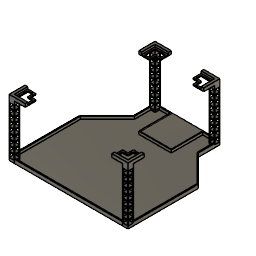
Maze solver chassis (Autodesk Fusion 360 design; units mm, degrees)
Autodesk Fusion 360 part; units mm, degrees
sketch "Sketch1" plane through (0, 0, 0) normal (0, 0, 1) x (1, 0, 0)
  line L0 (0, 0) -> (100, 0)
  line L1 (100, 0) -> (100, 60)
  line L2 (0, 0) -> (0, 60)
  line L3 (0, 60) -> (25, 85)
  line L4 (100, 60) -> (75, 85)
  line L5 (25, 85) -> (25, 100)
  line L6 (25, 100) -> (75, 100)
  line L7 (75, 100) -> (75, 85)
  line L8 (100, -5) -> (-5, -5)
  line L9 (-5, -5) -> (-5, 60)
  line L10 (105, 60) -> (105, -5)
  line L11 (105, -5) -> (100, -5)
  line L12 (25, 105) -> (75, 105)
  line L13 (75, 105) -> (80, 105)
  line L14 (80, 105) -> (80, 85)
  line L15 (80, 85) -> (105, 60)
  line L16 (25, 105) -> (20, 105)
  line L17 (20, 105) -> (20, 85)
  line L18 (20, 85) -> (-5, 60)
  line L19 (0, 0) -> (5, 0)
  line L20 (5, 5) -> (95, 5)
  line L21 (95, 5) -> (95, 60)
  line L22 (5, 60) -> (5, 5)
  line L23 (30, 95) -> (70, 95)
  line L24 (70, 95) -> (70, 85)
  line L25 (70, 85) -> (95, 60)
  line L26 (30, 95) -> (30, 85)
  line L27 (30, 85) -> (5, 60)
  dimension "d2" = 60
  dimension "d3" = 60
  dimension "d8" = 50
  dimension "d10" = 5
  dimension "d11" = 105
  dimension "d12" = 65
  dimension "d13" = 110
  constraint coincident L0.start L2.start
  constraint horizontal L0
  constraint coincident L0 L19.end
  measures "d2" distance of L0.end L1.end
  measures "d3" distance of L0.start L2.end
  measures "d8" distance of L5.end L6.end
  measures "d10" distance of L0.end L8.start
  measures "d11" distance of L8.start L8.end
  measures "d12" distance of L8.end L9.end
  measures "d13" distance of L9.end L10.start
sketch "Sketch2" plane through (0, 0, 0) normal (0, 0, 1) x (1, 0, 0)
  line L0 (102.5, 10) -> (105, 10)
  line L1 (105, 10) -> (105, -5)
  line L2 (105, -5) -> (90, -5)
  line L3 (90, -5) -> (90, -2.5)
  line L4 (-5, -5) -> (10, -5)
  line L5 (10, -5) -> (10, -2.5)
  line L6 (-2.5, 10) -> (-5, 10)
  line L7 (-5, 10) -> (-5, -5)
  line L8 (65, 102.5) -> (65, 105)
  line L9 (65, 105) -> (80, 105)
  line L10 (80, 105) -> (80, 90)
  line L11 (80, 90) -> (77.5, 90)
  line L12 (35, 102.5) -> (35, 105)
  line L13 (35, 105) -> (20, 105)
  line L14 (20, 105) -> (20, 95)
  line L15 (20, 95) -> (20, 90)
  line L16 (20, 90) -> (22.5, 90)
  line L17 (20, 90) -> (22.5, 90)
  line L18 (20, 90) -> (22.5, 90)
  line L19 (22.5, 90) -> (22.5, 102.5)
  line L20 (35, 102.5) -> (22.5, 102.5)
  line L21 (65, 102.5) -> (77.5, 102.5)
  line L22 (77.5, 102.5) -> (77.5, 90)
  line L23 (102.5, 10) -> (102.5, -2.5)
  line L24 (102.5, -2.5) -> (90, -2.5)
  line L25 (10, -2.5) -> (-2.5, -2.5)
  line L26 (-2.5, -2.5) -> (-2.5, 10)
  line L27 (35, 102.5) -> (35, 95)
  line L28 (30, 95) -> (35, 95)
  line L29 (30, 95) -> (30, 90)
  line L30 (30, 90) -> (22.5, 90)
  line L31 (65, 102.5) -> (65, 95)
  line L32 (65, 95) -> (70, 95)
  line L33 (70, 95) -> (70, 90)
  line L34 (70, 90) -> (77.5, 90)
  line L35 (102.5, 10) -> (95, 10)
  line L36 (95, 10) -> (95, 5)
  line L37 (95, 5) -> (90, 5)
  line L38 (90, 5) -> (90, -2.5)
  line L39 (-2.5, 10) -> (5, 10)
  line L40 (5, 10) -> (5, 5)
  line L41 (5, 5) -> (10, 5)
  line L42 (10, 5) -> (10, -2.5)
  line L43 (90, 5) -> (90, 3.5)
  line L44 (91.5, 3.5) -> (95, 3.5)
  line L45 (95, 5) -> (95, 10)
  line L46 (95, 10) -> (96.5, 10)
  line L47 (96.5, 8.5) -> (96.5, 3.5)
  line L48 (96.5, 3.5) -> (95, 3.5)
  line L49 (91.5, 3.5) -> (91.5, -1)
  line L50 (91.5, -1) -> (101, -1)
  line L51 (101, -1) -> (101, 8.5)
  line L52 (101, 8.5) -> (96.5, 8.5)
  line L53 (10, 5) -> (10, 3.5)
  line L54 (8.5, 3.5) -> (3.5, 3.5)
  line L55 (3.5, 3.5) -> (3.5, 8.5)
  line L56 (3.5, 8.5) -> (-1, 8.5)
  line L57 (-1, 8.5) -> (-1, -1)
  line L58 (-1, -1) -> (8.5, -1)
  line L59 (8.5, -1) -> (8.5, 3.5)
  line L60 (35, 102.5) -> (35, 101)
  line L61 (33.5, 101) -> (24, 101)
  line L62 (24, 101) -> (24, 91.5)
  line L63 (24, 91.5) -> (28.5, 91.5)
  line L64 (28.5, 91.5) -> (28.5, 96.5)
  line L65 (28.5, 96.5) -> (33.5, 96.5)
  line L66 (33.5, 96.5) -> (33.5, 101)
  line L67 (65, 102.5) -> (65, 101)
  line L68 (66.5, 101) -> (76, 101)
  line L69 (76, 101) -> (76, 91.5)
  line L70 (76, 91.5) -> (71.5, 91.5)
  line L71 (71.5, 91.5) -> (71.5, 96.5)
  line L72 (71.5, 96.5) -> (66.5, 96.5)
  line L73 (66.5, 96.5) -> (66.5, 101)
  dimension "d16" = 15
  dimension "d17" = 15
  constraint coincident L38 L43.end
  constraint coincident L35 L46.end
  constraint coincident L42 L53.end
  constraint coincident L31 L67.end
  measures "d16" distance of L4.start L4.end
  measures "d17" distance of L9.end L10.end
sketch "Sketch3" plane through (0, 0, 0) normal (0, 0, 1) x (1, 0, 0)
  line L0 (100, -5) -> (100, 0)
  line L1 (100, 0) -> (105, 0)
  line L2 (105, 0) -> (105, -5)
  line L3 (105, -5) -> (100, -5)
  line L4 (75, 100) -> (75, 105)
  line L5 (75, 105) -> (80, 105)
  line L6 (80, 105) -> (80, 100)
  line L7 (80, 100) -> (75, 100)
  line L8 (25, 100) -> (25, 105)
  line L9 (25, 105) -> (20, 105)
  line L10 (20, 105) -> (20, 100)
  line L11 (20, 100) -> (25, 100)
  line L12 (-5, -5) -> (0, -5)
  line L13 (0, -5) -> (0, 0)
  line L14 (0, 0) -> (-5, 0)
  line L15 (-5, 0) -> (-5, -5)
  constraint vertical L0
  constraint perpendicular L0 L1
  constraint perpendicular L1 L2
  constraint perpendicular L0 L3
  constraint perpendicular L1 L4
  constraint perpendicular L4 L5
  constraint perpendicular L5 L6
  constraint perpendicular L4 L7
  constraint perpendicular L5 L8
  constraint perpendicular L4 L9
  constraint perpendicular L9 L10
  constraint perpendicular L4 L11
  constraint perpendicular L4 L12
  constraint coincident L13.end L14.start
  constraint perpendicular L9 L13
  constraint perpendicular L13 L14
  constraint perpendicular L12 L15
sketch "Sketch4" plane through (0, 0, 0) normal (0, 0, 1) x (1, 0, 0)
  line L0 (-5, -5, -50) -> (-5, 105, -50)
  line L1 (-5, 105, -50) -> (105, 105, -50)
  line L2 (105, 105, -50) -> (105, -5, -50)
  line L3 (105, -5, -50) -> (-5, -5, -50)
extrude "Extrude1" add sketch "Sketch2" along normal blind 1 contours L0 L1 L2 L3 L23 L24 | L23 L24 L35 L36 L37 L38 L43 L45 L46 | L4 L5 L6 L7 L25 L26 | L25 L26 L39 L40 L41 L42 L53 | L8 L9 L10 L11 L21 L22 | L21 L22 L31 L32 L33 L34 L67 | L12 L13 L14 L15 L16 L17 L18 L19 L20 | L19 L20 L27 L28 L29 L30 L60 | L44 L47 L48 L49 L50 L51 L52 | L54 L55 L56 L57 L58 L59 | L61 L62 L63 L64 L65 L66 | L68 L69 L70 L71 L72 L73 makes body 1 at (-1.6667, 3.3333, 0) makes body 2 at (28.3333, 101.6667, 0) makes body 3 at (96.6667, -1.6667, 0) makes body 4 at (71.6667, 101.6667, 0)
extrude "Extrude2" add sketch "Sketch2" along normal blind 3 contours L0 L1 L2 L3 L23 L24 | L4 L5 L6 L7 L25 L26 | L8 L9 L10 L11 L21 L22 | L12 L13 L14 L15 L16 L17 L18 L19 L20 bodies 1 2 3 4
extrude "Extrude3" add sketch "Sketch3" against normal blind 50 bodies 1 2 3 4
extrude "Extrude4" add sketch "Sketch4" along normal blind 1 contours L0 L1 L2 L3 in plane through (0, 0, -50) normal (0, 0, 1) bodies 1 2 3 4
sketch "Sketch5" plane through (0, 0, 0) normal (0, 0, 1) x (1, 0, 0)
  line L0 (20, 85, -50) -> (-5, 60, -50)
  line L1 (20, 105, -50) -> (20, 85, -50)
  line L2 (25, 105, -50) -> (20, 105, -50)
  line L3 (25, 105, -50) -> (75, 105, -50)
  line L4 (75, 105, -50) -> (80, 105, -50)
  line L5 (80, 105, -50) -> (80, 85, -50)
  line L6 (80, 85, -50) -> (105, 60, -50)
  line L7 (105, 60, -50) -> (105, -5, -50)
  line L8 (105, -5, -50) -> (100, -5, -50)
  line L9 (100, -5, -50) -> (-5, -5, -50)
  line L10 (-5, -5, -50) -> (-5, 60, -50)
  dimension "d27" = 105
  dimension "d28" = 65
  dimension "d29" = 110
ref_plane "WorkPlane1" through (50, 50, -50) normal (0, 0, 1) x (1, 0, 0)
sketch "Sketch6" plane through (0, 0, -50) normal (0, 0, 1) x (1, 0, 0)
  line L0 (-5, 60) -> (-5, 105)
  line L1 (-5, 105) -> (20, 105)
  line L2 (20, 105) -> (20, 85)
  line L3 (20, 85) -> (-5, 60)
  line L4 (80, 105) -> (105, 105)
  line L5 (105, 105) -> (105, 60)
  line L6 (105, 60) -> (80, 85)
  line L7 (80, 85) -> (80, 105)
  constraint vertical L0
  constraint perpendicular L0 L1
  constraint perpendicular L1 L2
  constraint perpendicular L0 L4
  constraint perpendicular L4 L5
  constraint perpendicular L3 L6
  constraint perpendicular L4 L7
extrude "Extrude5" cut sketch "Sketch6" along normal blind 1 bodies 1
sketch "Sketch7" plane through (0, 0, -50) normal (0, 0, 1) x (1, 0, 0)
  line L0 (50, 105) -> (65, 105)
  line L1 (65, 105) -> (65, 75)
  line L2 (65, 75) -> (35, 75)
  line L3 (35, 75) -> (35, 105)
  line L4 (35, 105) -> (50, 105)
  dimension "d33" = 15
  dimension "d34" = 30
  dimension "d35" = 30
  dimension "d36" = 30
  constraint horizontal L0
  constraint perpendicular L0 L1
  constraint perpendicular L1 L2
  constraint perpendicular L0 L3
  measures "d33" distance of L0.start L0.end
  measures "d34" distance of L0.end L1.end
  measures "d35" distance of L1.end L2.end
  measures "d36" distance of L2.end L3.end
extrude "Extrude6" add sketch "Sketch7" along normal blind 10 bodies 1
extrude "Extrude7" cut sketch "Sketch7" along normal blind 9 bodies 1 makes body 5 at (45, 95, -41)
sketch "Sketch8" plane through (0, 0, -50) normal (0, 0, 1) x (1, 0, 0)
  line L0 (35, 105) -> (36, 105)
  line L1 (36, 105) -> (36, 76)
  line L2 (36, 76) -> (64, 76)
  line L3 (64, 76) -> (64, 105)
  line L4 (35, 105) -> (36, 105)
  line L5 (64, 105) -> (65, 105)
  line L6 (36, 105) -> (35, 105)
  line L7 (35, 105) -> (35, 75)
  line L8 (35, 75) -> (65, 75)
  line L9 (65, 75) -> (65, 105)
  line L10 (64, 105) -> (36, 105)
  constraint perpendicular L1 L6
  constraint perpendicular L6 L7
  constraint perpendicular L1 L8
  constraint perpendicular L5 L9
  constraint perpendicular L1 L10
extrude "Extrude8" add sketch "Sketch8" along normal blind 10 contours L0 L1 L2 L3 L4 L5 L6 L7 L8 L9 bodies 1 5
sketch "Sketch9" plane through (0, 0, 0) normal (1, 0, 0) x (0, 1, 0)
  line L0 (10, -50) -> (10, -65)
  circle A0 centre (10, -57.5) radius 25
  line L1 (10, -82.5) -> (100, -82.5)
  line L2 (100, -82.5) -> (100, -47.5)
  line L3 (105, -50) -> (105, -47.5)
  line L4 (105, -47.5) -> (75, -47.5)
  dimension "d43" = 15
  dimension "d45" = 35
  dimension "d46" = 2.5
  dimension "d47" = 30
  constraint coincident A0 L1.start
  constraint tangent A0 L1
  constraint perpendicular L0 L1
  constraint perpendicular L1 L2
  constraint vertical L3
  constraint perpendicular L3 L4
  measures "d43" distance of L0.start L0.end
  measures "d45" distance of L1.end L2.end
  measures "d46" distance of L3.start L3.end
  measures "d47" distance of L3.end L4.end
sketch "Sketch10" plane through (0, 105, 0) normal (0, 1, 0) x (-1, 0, 0)
  line L0 (-65, -49) -> (-75, -49)
  line L1 (-75, -49) -> (-75, 0)
  line L2 (-75, 0) -> (-65, 0)
  line L3 (-65, 0) -> (-65, 3)
  line L4 (-65, 3) -> (-80, 3)
  line L5 (-80, 3) -> (-80, -50)
  line L6 (-80, -50) -> (-64, -50)
  line L7 (-64, -50) -> (-64, -41)
  line L8 (-64, -41) -> (-36, -41)
  line L9 (-36, -41) -> (-36, -50)
  line L10 (-36, -50) -> (-20, -50)
  line L11 (-20, -50) -> (-20, 3)
  line L12 (-20, 3) -> (-35, 3)
  line L13 (-35, 3) -> (-35, 0)
  line L14 (-35, 0) -> (-25, 0)
  line L15 (-25, 0) -> (-25, -49)
  line L16 (-25, -49) -> (-35, -49)
  line L17 (-35, -49) -> (-35, -40)
  line L18 (-35, -40) -> (-65, -40)
  line L19 (-65, -40) -> (-65, -49)
  line L20 (0, -47.5) -> (-100, -47.5)
  constraint perpendicular L5 L20
extrude "Extrude9" cut 1 faces at (45, 95, -40) along direction (0, 0, -1) blind 7.5 on bodies 1 bodies 1
extrude "Extrude10" add sketch "Sketch7" along normal blind 3.5 bodies 1
extrude "Extrude11" cut sketch "Sketch8" along normal blind 3 contours L1 L2 L3 L10 bodies 1
extrude "Extrude12" cut sketch "Sketch2" along normal blind 2 contours L44 L47 L48 L49 L50 L51 L52 | L54 L55 L56 L57 L58 L59 | L61 L62 L63 L64 L65 L66 | L68 L69 L70 L71 L72 L73 bodies 1
sketch "Sketch11" plane through (-5, 0, 0) normal (-1, 0, 0) x (0, -1, 0)
  line L0 (-60, -49) -> (-60, -50)
  line L1 (-60, -50) -> (5, -50)
  line L2 (5, -50) -> (5, 3)
  line L3 (5, 3) -> (-10, 3)
  line L4 (-10, 3) -> (-10, 0)
  line L5 (-10, 0) -> (0, 0)
  line L6 (0, 0) -> (0, -49)
  line L7 (0, -49) -> (-60, -49)
  line L8 (5, -50) -> (2.5, -50)
  line L9 (4.5, -47.5) -> (0.5, -47.5)
  line L10 (0.5, -47.5) -> (0.5, -43.5)
  line L11 (0.5, -43.5) -> (4.5, -43.5)
  line L12 (4.5, -43.5) -> (4.5, -47.5)
  line L13 (4.5, -47.5) -> (0.5, -43.5) construction
  line L14 (0.5, -38.5) -> (4.5, -38.5)
  line L15 (0.5, -42.5) -> (0.5, -38.5)
  line L16 (4.5, -42.5) -> (0.5, -38.5) construction
  line L17 (4.5, -38.5) -> (4.5, -42.5)
  line L18 (4.5, -42.5) -> (0.5, -42.5)
  line L19 (4.5, -32.5) -> (0.5, -32.5)
  line L20 (0.5, -28.5) -> (4.5, -28.5)
  line L21 (4.5, -28.5) -> (4.5, -32.5)
  line L22 (4.5, -37.5) -> (0.5, -37.5)
  line L23 (4.5, -32.5) -> (0.5, -28.5) construction
  line L24 (0.5, -33.5) -> (4.5, -33.5)
  line L25 (4.5, -33.5) -> (4.5, -37.5)
  line L26 (0.5, -32.5) -> (0.5, -28.5)
  line L27 (0.5, -37.5) -> (0.5, -33.5)
  line L28 (4.5, -37.5) -> (0.5, -33.5) construction
  line L29 (4.5, -22.5) -> (0.5, -22.5)
  line L30 (0.5, -17.5) -> (0.5, -13.5)
  line L31 (0.5, -27.5) -> (0.5, -23.5)
  line L32 (4.5, -12.5) -> (0.5, -8.5) construction
  line L33 (0.5, -13.5) -> (4.5, -13.5)
  line L34 (0.5, -12.5) -> (0.5, -8.5)
  line L35 (4.5, -12.5) -> (0.5, -12.5)
  line L36 (0.5, -8.5) -> (4.5, -8.5)
  line L37 (0.5, -18.5) -> (4.5, -18.5)
  line L38 (4.5, -17.5) -> (0.5, -17.5)
  line L39 (4.5, -27.5) -> (0.5, -23.5) construction
  line L40 (5, -30) -> (2.5, -30)
  line L41 (0.5, -22.5) -> (0.5, -18.5)
  line L42 (4.5, -18.5) -> (4.5, -22.5)
  line L43 (4.5, -23.5) -> (4.5, -27.5)
  line L44 (4.5, -27.5) -> (0.5, -27.5)
  line L45 (4.5, -22.5) -> (0.5, -18.5) construction
  line L46 (0.5, -23.5) -> (4.5, -23.5)
  line L47 (4.5, -13.5) -> (4.5, -17.5)
  line L48 (4.5, -8.5) -> (4.5, -12.5)
  line L49 (4.5, -17.5) -> (0.5, -13.5) construction
  line L50 (0.5, -7.5) -> (0.5, -3.5)
  line L51 (4.5, -7.5) -> (0.5, -7.5)
  line L52 (4.5, -7.5) -> (0.5, -3.5) construction
  line L53 (4.5, -3.5) -> (4.5, -7.5)
  line L54 (0.5, -3.5) -> (4.5, -3.5)
  line L55 (0.5, -23.5) -> (4.5, -23.5)
  line L56 (0.5, -13.5) -> (4.5, -13.5)
  line L57 (4.5, -38.5) -> (4.5, -42.5)
  line L58 (4.5, -3.5) -> (4.5, -7.5)
  line L59 (4.5, -43.5) -> (4.5, -47.5)
  line L60 (0.5, -7.5) -> (0.5, -3.5)
  line L61 (4.5, -7.5) -> (0.5, -3.5) construction
  line L62 (4.5, -22.5) -> (0.5, -22.5)
  line L63 (4.5, -47.5) -> (0.5, -47.5)
  line L64 (4.5, -12.5) -> (0.5, -8.5) construction
  line L65 (4.5, -12.5) -> (0.5, -12.5)
  line L66 (0.5, -42.5) -> (0.5, -38.5)
  line L67 (4.5, -32.5) -> (0.5, -32.5)
  line L68 (4.5, -42.5) -> (0.5, -42.5)
  line L69 (4.5, -42.5) -> (0.5, -38.5) construction
  line L70 (0.5, -47.5) -> (0.5, -43.5)
  line L71 (5, -50) -> (2.5, -50)
  line L72 (4.5, -28.5) -> (4.5, -32.5)
  line L73 (0.5, -43.5) -> (4.5, -43.5)
  line L74 (0.5, -37.5) -> (0.5, -33.5)
  line L75 (0.5, -3.5) -> (4.5, -3.5)
  line L76 (4.5, -7.5) -> (0.5, -7.5)
  line L77 (0.5, -8.5) -> (4.5, -8.5)
  line L78 (4.5, -47.5) -> (0.5, -43.5) construction
  line L79 (4.5, -8.5) -> (4.5, -12.5)
  line L80 (0.5, -12.5) -> (0.5, -8.5)
  line L81 (0.5, -38.5) -> (4.5, -38.5)
  line L82 (0.5, -18.5) -> (4.5, -18.5)
  line L83 (0.5, -22.5) -> (0.5, -18.5)
  line L84 (4.5, -33.5) -> (4.5, -37.5)
  line L85 (4.5, -23.5) -> (4.5, -27.5)
  line L86 (0.5, -28.5) -> (4.5, -28.5)
  line L87 (4.5, -37.5) -> (0.5, -37.5)
  line L88 (4.5, -18.5) -> (4.5, -22.5)
  line L89 (4.5, -27.5) -> (0.5, -27.5)
  line L90 (0.5, -32.5) -> (0.5, -28.5)
  line L91 (4.5, -32.5) -> (0.5, -28.5) construction
  line L92 (4.5, -27.5) -> (0.5, -23.5) construction
  line L93 (4.5, -22.5) -> (0.5, -18.5) construction
  line L94 (4.5, -17.5) -> (0.5, -17.5)
  line L95 (4.5, -37.5) -> (0.5, -33.5) construction
  line L96 (5, -30) -> (2.5, -30)
  line L97 (0.5, -33.5) -> (4.5, -33.5)
  line L98 (0.5, -27.5) -> (0.5, -23.5)
  line L99 (4.5, -13.5) -> (4.5, -17.5)
  line L100 (0.5, -17.5) -> (0.5, -13.5)
  line L101 (4.5, -17.5) -> (0.5, -13.5) construction
  line L102 (-104.5, -23.5) -> (-100.5, -23.5)
  line L103 (-104.5, -13.5) -> (-100.5, -13.5)
  line L104 (-100.5, -38.5) -> (-100.5, -42.5)
  line L105 (-100.5, -3.5) -> (-100.5, -7.5)
  line L106 (-100.5, -43.5) -> (-100.5, -47.5)
  line L107 (-104.5, -7.5) -> (-104.5, -3.5)
  line L108 (-100.5, -7.5) -> (-104.5, -3.5) construction
  line L109 (-100.5, -22.5) -> (-104.5, -22.5)
  line L110 (-100.5, -47.5) -> (-104.5, -47.5)
  line L111 (-100.5, -12.5) -> (-104.5, -8.5) construction
  line L112 (-100.5, -12.5) -> (-104.5, -12.5)
  line L113 (-104.5, -42.5) -> (-104.5, -38.5)
  line L114 (-100.5, -32.5) -> (-104.5, -32.5)
  line L115 (-100.5, -42.5) -> (-104.5, -42.5)
  line L116 (-100.5, -42.5) -> (-104.5, -38.5) construction
  line L117 (-104.5, -47.5) -> (-104.5, -43.5)
  line L118 (-100, -50) -> (-102.5, -50)
  line L119 (-100.5, -28.5) -> (-100.5, -32.5)
  line L120 (-104.5, -43.5) -> (-100.5, -43.5)
  line L121 (-104.5, -37.5) -> (-104.5, -33.5)
  line L122 (-104.5, -3.5) -> (-100.5, -3.5)
  line L123 (-100.5, -7.5) -> (-104.5, -7.5)
  line L124 (-104.5, -8.5) -> (-100.5, -8.5)
  line L125 (-100.5, -47.5) -> (-104.5, -43.5) construction
  line L126 (-100.5, -8.5) -> (-100.5, -12.5)
  line L127 (-104.5, -12.5) -> (-104.5, -8.5)
  line L128 (-104.5, -38.5) -> (-100.5, -38.5)
  line L129 (-104.5, -18.5) -> (-100.5, -18.5)
  line L130 (-104.5, -22.5) -> (-104.5, -18.5)
  line L131 (-100.5, -33.5) -> (-100.5, -37.5)
  line L132 (-100.5, -23.5) -> (-100.5, -27.5)
  line L133 (-104.5, -28.5) -> (-100.5, -28.5)
  line L134 (-100.5, -37.5) -> (-104.5, -37.5)
  line L135 (-100.5, -18.5) -> (-100.5, -22.5)
  line L136 (-100.5, -27.5) -> (-104.5, -27.5)
  line L137 (-104.5, -32.5) -> (-104.5, -28.5)
  line L138 (-100.5, -32.5) -> (-104.5, -28.5) construction
  line L139 (-100.5, -27.5) -> (-104.5, -23.5) construction
  line L140 (-100.5, -22.5) -> (-104.5, -18.5) construction
  line L141 (-100.5, -17.5) -> (-104.5, -17.5)
  line L142 (-100.5, -37.5) -> (-104.5, -33.5) construction
  line L143 (-100, -30) -> (-102.5, -30)
  line L144 (-104.5, -33.5) -> (-100.5, -33.5)
  line L145 (-104.5, -27.5) -> (-104.5, -23.5)
  line L146 (-100.5, -13.5) -> (-100.5, -17.5)
  line L147 (-104.5, -17.5) -> (-104.5, -13.5)
  line L148 (-100.5, -17.5) -> (-104.5, -13.5) construction
  point P0 (2.5, -45.5)
  point P1 (2.5, -40.5)
  point P2 (2.5, -30.5)
  point P3 (2.5, -35.5)
  point P4 (2.5, -20.5)
  point P5 (2.5, -10.5)
  point P6 (2.5, -15.5)
  point P7 (2.5, -25.5)
  point P8 (0, -29)
  point P9 (2.5, -5.5)
  point P10 (2.5, -5.5)
  point P11 (2.5, -40.5)
  point P12 (2.5, -20.5)
  point P13 (2.5, -30.5)
  point P14 (2.5, -35.5)
  point P15 (2.5, -15.5)
  point P16 (2.5, -25.5)
  point P17 (0, -29)
  point P18 (2.5, -10.5)
  point P19 (2.5, -45.5)
  point P20 (5, -50)
  point P21 (0, -49)
  point P22 (-102.5, -5.5)
  point P23 (-102.5, -40.5)
  point P24 (-102.5, -20.5)
  point P25 (-102.5, -30.5)
  point P26 (-102.5, -35.5)
  point P27 (-102.5, -15.5)
  point P28 (-102.5, -25.5)
  point P29 (-105, -29)
  point P30 (-102.5, -10.5)
  point P31 (-102.5, -45.5)
  point P32 (-100, -50)
  point P33 (-105, -49)
  dimension "d74" = 2.5
  dimension "d79" = 2.5
  dimension "d80" = 2.5
  dimension "d81" = 2.5
  dimension "d82" = 2.5
  dimension "d83" = 2.5
  constraint coincident P20 L1.end
  constraint coincident L1 L8.end
  constraint horizontal L9
  constraint coincident L13 P19
  constraint horizontal L18
  constraint coincident P11 L16
  constraint horizontal L22
  constraint coincident P14 L28
  constraint horizontal L19
  constraint coincident P13 L23
  constraint horizontal L44
  constraint coincident P16 L39
  constraint horizontal L29
  constraint coincident P12 L45
  constraint horizontal L38
  constraint coincident P15 L49
  constraint horizontal L35
  constraint coincident P18 L32
  constraint horizontal L51
  constraint coincident P10 L52
  constraint horizontal L63
  constraint coincident P19 L78
  constraint horizontal L68
  constraint coincident P11 L69
  constraint horizontal L87
  constraint coincident P14 L95
  constraint horizontal L67
  constraint coincident P13 L91
  constraint horizontal L89
  constraint coincident P16 L92
  constraint horizontal L62
  constraint coincident P12 L93
  constraint horizontal L94
  constraint coincident P15 L101
  constraint horizontal L65
  constraint coincident P18 L64
  constraint horizontal L76
  constraint coincident P10 L61
  constraint coincident P32 L118.start
  constraint horizontal L110
  constraint coincident P31 L125
  constraint horizontal L115
  constraint coincident P23 L116
  constraint horizontal L134
  constraint coincident P26 L142
  constraint horizontal L114
  constraint coincident P25 L138
  constraint horizontal L136
  constraint coincident P28 L139
  constraint horizontal L109
  constraint coincident P24 L140
  constraint horizontal L141
  constraint coincident P27 L148
  constraint horizontal L112
  constraint coincident P30 L111
  constraint horizontal L123
  constraint coincident P22 L108
  measures "d74" distance of P20 L8.end
  measures "d79" distance of L40.start L40.end
  measures "d80" distance of P20 L8.end
  measures "d81" distance of L40.start L40.end
  measures "d82" distance of P32 L118.end
  measures "d83" distance of L143.start L143.end
extrude "Extrude13" cut sketch "Sketch11" against normal blind 120 contours L9 L10 L11 L12 L59 L63 L70 L73 | L14 L15 L17 L18 L57 L66 L68 L81 | L19 L20 L21 L26 L67 L72 L86 L90 | L22 L24 L25 L27 L74 L84 L87 L97 | L29 L37 L41 L42 L62 L82 L83 L88 | L30 L33 L38 L47 L56 L94 L99 L100 | L31 L43 L44 L46 L55 L85 L89 L98 | L34 L35 L36 L48 L65 L77 L79 L80 | L50 L51 L53 L54 L58 L60 L75 L76 | L102 L132 L136 L145 | L103 L141 L146 L147 | L104 L113 L115 L128 | L105 L107 L122 L123 | L109 L129 L130 L135 | L112 L124 L126 L127 | L114 L119 L133 L137 | L121 L131 L134 L144 bodies 1
sketch "Sketch12" plane through (0, -5, 0) normal (0, -1, 0) x (1, 0, 0)
  line L0 (0, -49) -> (0, 0)
  line L1 (0, 0) -> (10, 0)
  line L2 (10, 0) -> (10, 3)
  line L3 (10, 3) -> (-5, 3)
  line L4 (-5, 3) -> (-5, -50)
  line L5 (-5, -50) -> (0, -50)
  line L6 (0, -50) -> (0, -49)
  line L7 (-4.5, -23.5) -> (-0.5, -23.5)
  line L8 (-4.5, -13.5) -> (-0.5, -13.5)
  line L9 (-0.5, -38.5) -> (-0.5, -42.5)
  line L10 (-0.5, -3.5) -> (-0.5, -7.5)
  line L11 (-0.5, -43.5) -> (-0.5, -47.5)
  line L12 (-4.5, -7.5) -> (-4.5, -3.5)
  line L13 (-0.5, -7.5) -> (-4.5, -3.5) construction
  line L14 (-0.5, -22.5) -> (-4.5, -22.5)
  line L15 (-0.5, -47.5) -> (-4.5, -47.5)
  line L16 (-0.5, -12.5) -> (-4.5, -8.5) construction
  line L17 (-0.5, -12.5) -> (-4.5, -12.5)
  line L18 (-4.5, -42.5) -> (-4.5, -38.5)
  line L19 (-0.5, -32.5) -> (-4.5, -32.5)
  line L20 (-0.5, -42.5) -> (-4.5, -42.5)
  line L21 (-0.5, -42.5) -> (-4.5, -38.5) construction
  line L22 (-4.5, -47.5) -> (-4.5, -43.5)
  line L23 (0, -50) -> (-2.5, -50)
  line L24 (-0.5, -28.5) -> (-0.5, -32.5)
  line L25 (-4.5, -43.5) -> (-0.5, -43.5)
  line L26 (-4.5, -37.5) -> (-4.5, -33.5)
  line L27 (-4.5, -3.5) -> (-0.5, -3.5)
  line L28 (-0.5, -7.5) -> (-4.5, -7.5)
  line L29 (-4.5, -8.5) -> (-0.5, -8.5)
  line L30 (-0.5, -47.5) -> (-4.5, -43.5) construction
  line L31 (-0.5, -8.5) -> (-0.5, -12.5)
  line L32 (-4.5, -12.5) -> (-4.5, -8.5)
  line L33 (-4.5, -38.5) -> (-0.5, -38.5)
  line L34 (-4.5, -18.5) -> (-0.5, -18.5)
  line L35 (-4.5, -22.5) -> (-4.5, -18.5)
  line L36 (-0.5, -33.5) -> (-0.5, -37.5)
  line L37 (-0.5, -23.5) -> (-0.5, -27.5)
  line L38 (-4.5, -28.5) -> (-0.5, -28.5)
  line L39 (-0.5, -37.5) -> (-4.5, -37.5)
  line L40 (-0.5, -18.5) -> (-0.5, -22.5)
  line L41 (-0.5, -27.5) -> (-4.5, -27.5)
  line L42 (-4.5, -32.5) -> (-4.5, -28.5)
  line L43 (-0.5, -32.5) -> (-4.5, -28.5) construction
  line L44 (-0.5, -27.5) -> (-4.5, -23.5) construction
  line L45 (-0.5, -22.5) -> (-4.5, -18.5) construction
  line L46 (-0.5, -17.5) -> (-4.5, -17.5)
  line L47 (-0.5, -37.5) -> (-4.5, -33.5) construction
  line L48 (0, -30) -> (-2.5, -30)
  line L49 (-4.5, -33.5) -> (-0.5, -33.5)
  line L50 (-4.5, -27.5) -> (-4.5, -23.5)
  line L51 (-0.5, -13.5) -> (-0.5, -17.5)
  line L52 (-4.5, -17.5) -> (-4.5, -13.5)
  line L53 (-0.5, -17.5) -> (-4.5, -13.5) construction
  point P0 (-2.5, -5.5)
  point P1 (-2.5, -40.5)
  point P2 (-2.5, -20.5)
  point P3 (-2.5, -30.5)
  point P4 (-2.5, -35.5)
  point P5 (-2.5, -15.5)
  point P6 (-2.5, -25.5)
  point P7 (-5, -29)
  point P8 (-2.5, -10.5)
  point P9 (-2.5, -45.5)
  point P10 (0, -50)
  point P11 (-5, -49)
  dimension "d86" = 2.5
  dimension "d87" = 2.5
  constraint coincident P10 L5.end
  constraint horizontal L15
  constraint coincident P9 L30
  constraint horizontal L20
  constraint coincident P1 L21
  constraint horizontal L39
  constraint coincident P4 L47
  constraint horizontal L19
  constraint coincident P3 L43
  constraint horizontal L41
  constraint coincident P6 L44
  constraint horizontal L14
  constraint coincident P2 L45
  constraint horizontal L46
  constraint coincident P5 L53
  constraint horizontal L17
  constraint coincident P8 L16
  constraint horizontal L28
  constraint coincident P0 L13
  measures "d86" distance of P10 L23.end
  measures "d87" distance of L48.start L48.end
sketch "Sketch13" plane through (0, -5, 0) normal (0, -1, 0) x (1, 0, 0)
  line L0 (105, -50) -> (105, 3)
  line L1 (105, 3) -> (90, 3)
  line L2 (90, 3) -> (90, 0)
  line L3 (90, 0) -> (100, 0)
  line L4 (100, 0) -> (100, -49)
  line L5 (100, -49) -> (100, -50)
  line L6 (100, -50) -> (105, -50)
  line L7 (100.5, -23.5) -> (104.5, -23.5)
  line L8 (100.5, -13.5) -> (104.5, -13.5)
  line L9 (104.5, -38.5) -> (104.5, -42.5)
  line L10 (104.5, -3.5) -> (104.5, -7.5)
  line L11 (104.5, -43.5) -> (104.5, -47.5)
  line L12 (100.5, -7.5) -> (100.5, -3.5)
  line L13 (104.5, -7.5) -> (100.5, -3.5) construction
  line L14 (104.5, -22.5) -> (100.5, -22.5)
  line L15 (104.5, -47.5) -> (100.5, -47.5)
  line L16 (104.5, -12.5) -> (100.5, -8.5) construction
  line L17 (104.5, -12.5) -> (100.5, -12.5)
  line L18 (100.5, -42.5) -> (100.5, -38.5)
  line L19 (104.5, -32.5) -> (100.5, -32.5)
  line L20 (104.5, -42.5) -> (100.5, -42.5)
  line L21 (104.5, -42.5) -> (100.5, -38.5) construction
  line L22 (100.5, -47.5) -> (100.5, -43.5)
  line L23 (105, -50) -> (102.5, -50)
  line L24 (104.5, -28.5) -> (104.5, -32.5)
  line L25 (100.5, -43.5) -> (104.5, -43.5)
  line L26 (100.5, -37.5) -> (100.5, -33.5)
  line L27 (100.5, -3.5) -> (104.5, -3.5)
  line L28 (104.5, -7.5) -> (100.5, -7.5)
  line L29 (100.5, -8.5) -> (104.5, -8.5)
  line L30 (104.5, -47.5) -> (100.5, -43.5) construction
  line L31 (104.5, -8.5) -> (104.5, -12.5)
  line L32 (100.5, -12.5) -> (100.5, -8.5)
  line L33 (100.5, -38.5) -> (104.5, -38.5)
  line L34 (100.5, -18.5) -> (104.5, -18.5)
  line L35 (100.5, -22.5) -> (100.5, -18.5)
  line L36 (104.5, -33.5) -> (104.5, -37.5)
  line L37 (104.5, -23.5) -> (104.5, -27.5)
  line L38 (100.5, -28.5) -> (104.5, -28.5)
  line L39 (104.5, -37.5) -> (100.5, -37.5)
  line L40 (104.5, -18.5) -> (104.5, -22.5)
  line L41 (104.5, -27.5) -> (100.5, -27.5)
  line L42 (100.5, -32.5) -> (100.5, -28.5)
  line L43 (104.5, -32.5) -> (100.5, -28.5) construction
  line L44 (104.5, -27.5) -> (100.5, -23.5) construction
  line L45 (104.5, -22.5) -> (100.5, -18.5) construction
  line L46 (104.5, -17.5) -> (100.5, -17.5)
  line L47 (104.5, -37.5) -> (100.5, -33.5) construction
  line L48 (105, -30) -> (102.5, -30)
  line L49 (100.5, -33.5) -> (104.5, -33.5)
  line L50 (100.5, -27.5) -> (100.5, -23.5)
  line L51 (104.5, -13.5) -> (104.5, -17.5)
  line L52 (100.5, -17.5) -> (100.5, -13.5)
  line L53 (104.5, -17.5) -> (100.5, -13.5) construction
  point P0 (102.5, -5.5)
  point P1 (102.5, -40.5)
  point P2 (102.5, -20.5)
  point P3 (102.5, -30.5)
  point P4 (102.5, -35.5)
  point P5 (102.5, -15.5)
  point P6 (102.5, -25.5)
  point P7 (100, -29)
  point P8 (102.5, -10.5)
  point P9 (102.5, -45.5)
  point P10 (105, -50)
  point P11 (100, -49)
  dimension "d88" = 2.5
  dimension "d89" = 2.5
  constraint coincident P10 L0.start
  constraint horizontal L15
  constraint coincident P9 L30
  constraint horizontal L20
  constraint coincident P1 L21
  constraint horizontal L39
  constraint coincident P4 L47
  constraint horizontal L19
  constraint coincident P3 L43
  constraint horizontal L41
  constraint coincident P6 L44
  constraint horizontal L14
  constraint coincident P2 L45
  constraint horizontal L46
  constraint coincident P5 L53
  constraint horizontal L17
  constraint coincident P8 L16
  constraint horizontal L28
  constraint coincident P0 L13
  measures "d88" distance of P10 L23.end
  measures "d89" distance of L48.start L48.end
sketch "Sketch14" plane through (0, 100, 0) normal (0, -1, 0) x (1, 0, 0)
  line L0 (75, -49) -> (80, -49)
  line L1 (80, -49) -> (80, 0)
  line L2 (80, 0) -> (76, 0)
  line L3 (76, 0) -> (75, 0)
  line L4 (75, 0) -> (75, -49)
  line L5 (75.5, -23.5) -> (79.5, -23.5)
  line L6 (75.5, -13.5) -> (79.5, -13.5)
  line L7 (79.5, -38.5) -> (79.5, -42.5)
  line L8 (79.5, -3.5) -> (79.5, -7.5)
  line L9 (79.5, -43.5) -> (79.5, -47.5)
  line L10 (75.5, -7.5) -> (75.5, -3.5)
  line L11 (79.5, -7.5) -> (75.5, -3.5) construction
  line L12 (79.5, -22.5) -> (75.5, -22.5)
  line L13 (79.5, -47.5) -> (75.5, -47.5)
  line L14 (79.5, -12.5) -> (75.5, -8.5) construction
  line L15 (79.5, -12.5) -> (75.5, -12.5)
  line L16 (75.5, -42.5) -> (75.5, -38.5)
  line L17 (79.5, -32.5) -> (75.5, -32.5)
  line L18 (79.5, -42.5) -> (75.5, -42.5)
  line L19 (79.5, -42.5) -> (75.5, -38.5) construction
  line L20 (75.5, -47.5) -> (75.5, -43.5)
  line L21 (80, -50) -> (77.5, -50)
  line L22 (79.5, -28.5) -> (79.5, -32.5)
  line L23 (75.5, -43.5) -> (79.5, -43.5)
  line L24 (75.5, -37.5) -> (75.5, -33.5)
  line L25 (75.5, -3.5) -> (79.5, -3.5)
  line L26 (79.5, -7.5) -> (75.5, -7.5)
  line L27 (75.5, -8.5) -> (79.5, -8.5)
  line L28 (79.5, -47.5) -> (75.5, -43.5) construction
  line L29 (79.5, -8.5) -> (79.5, -12.5)
  line L30 (75.5, -12.5) -> (75.5, -8.5)
  line L31 (75.5, -38.5) -> (79.5, -38.5)
  line L32 (75.5, -18.5) -> (79.5, -18.5)
  line L33 (75.5, -22.5) -> (75.5, -18.5)
  line L34 (79.5, -33.5) -> (79.5, -37.5)
  line L35 (79.5, -23.5) -> (79.5, -27.5)
  line L36 (75.5, -28.5) -> (79.5, -28.5)
  line L37 (79.5, -37.5) -> (75.5, -37.5)
  line L38 (79.5, -18.5) -> (79.5, -22.5)
  line L39 (79.5, -27.5) -> (75.5, -27.5)
  line L40 (75.5, -32.5) -> (75.5, -28.5)
  line L41 (79.5, -32.5) -> (75.5, -28.5) construction
  line L42 (79.5, -27.5) -> (75.5, -23.5) construction
  line L43 (79.5, -22.5) -> (75.5, -18.5) construction
  line L44 (79.5, -17.5) -> (75.5, -17.5)
  line L45 (79.5, -37.5) -> (75.5, -33.5) construction
  line L46 (80, -30) -> (77.5, -30)
  line L47 (75.5, -33.5) -> (79.5, -33.5)
  line L48 (75.5, -27.5) -> (75.5, -23.5)
  line L49 (79.5, -13.5) -> (79.5, -17.5)
  line L50 (75.5, -17.5) -> (75.5, -13.5)
  line L51 (79.5, -17.5) -> (75.5, -13.5) construction
  line L52 (20.5, -23.5) -> (24.5, -23.5)
  line L53 (20.5, -13.5) -> (24.5, -13.5)
  line L54 (24.5, -38.5) -> (24.5, -42.5)
  line L55 (24.5, -3.5) -> (24.5, -7.5)
  line L56 (24.5, -43.5) -> (24.5, -47.5)
  line L57 (20.5, -7.5) -> (20.5, -3.5)
  line L58 (24.5, -7.5) -> (20.5, -3.5) construction
  line L59 (24.5, -22.5) -> (20.5, -22.5)
  line L60 (24.5, -47.5) -> (20.5, -47.5)
  line L61 (24.5, -12.5) -> (20.5, -8.5) construction
  line L62 (24.5, -12.5) -> (20.5, -12.5)
  line L63 (20.5, -42.5) -> (20.5, -38.5)
  line L64 (24.5, -32.5) -> (20.5, -32.5)
  line L65 (24.5, -42.5) -> (20.5, -42.5)
  line L66 (24.5, -42.5) -> (20.5, -38.5) construction
  line L67 (20.5, -47.5) -> (20.5, -43.5)
  line L68 (25, -50) -> (22.5, -50)
  line L69 (24.5, -28.5) -> (24.5, -32.5)
  line L70 (20.5, -43.5) -> (24.5, -43.5)
  line L71 (20.5, -37.5) -> (20.5, -33.5)
  line L72 (20.5, -3.5) -> (24.5, -3.5)
  line L73 (24.5, -7.5) -> (20.5, -7.5)
  line L74 (20.5, -8.5) -> (24.5, -8.5)
  line L75 (24.5, -47.5) -> (20.5, -43.5) construction
  line L76 (24.5, -8.5) -> (24.5, -12.5)
  line L77 (20.5, -12.5) -> (20.5, -8.5)
  line L78 (20.5, -38.5) -> (24.5, -38.5)
  line L79 (20.5, -18.5) -> (24.5, -18.5)
  line L80 (20.5, -22.5) -> (20.5, -18.5)
  line L81 (24.5, -33.5) -> (24.5, -37.5)
  line L82 (24.5, -23.5) -> (24.5, -27.5)
  line L83 (20.5, -28.5) -> (24.5, -28.5)
  line L84 (24.5, -37.5) -> (20.5, -37.5)
  line L85 (24.5, -18.5) -> (24.5, -22.5)
  line L86 (24.5, -27.5) -> (20.5, -27.5)
  line L87 (20.5, -32.5) -> (20.5, -28.5)
  line L88 (24.5, -32.5) -> (20.5, -28.5) construction
  line L89 (24.5, -27.5) -> (20.5, -23.5) construction
  line L90 (24.5, -22.5) -> (20.5, -18.5) construction
  line L91 (24.5, -17.5) -> (20.5, -17.5)
  line L92 (24.5, -37.5) -> (20.5, -33.5) construction
  line L93 (25, -30) -> (22.5, -30)
  line L94 (20.5, -33.5) -> (24.5, -33.5)
  line L95 (20.5, -27.5) -> (20.5, -23.5)
  line L96 (24.5, -13.5) -> (24.5, -17.5)
  line L97 (20.5, -17.5) -> (20.5, -13.5)
  line L98 (24.5, -17.5) -> (20.5, -13.5) construction
  point P0 (77.5, -5.5)
  point P1 (77.5, -40.5)
  point P2 (77.5, -20.5)
  point P3 (77.5, -30.5)
  point P4 (77.5, -35.5)
  point P5 (77.5, -15.5)
  point P6 (77.5, -25.5)
  point P7 (75, -29)
  point P8 (77.5, -10.5)
  point P9 (77.5, -45.5)
  point P10 (80, -50)
  point P11 (75, -49)
  point P12 (22.5, -5.5)
  point P13 (22.5, -40.5)
  point P14 (22.5, -20.5)
  point P15 (22.5, -30.5)
  point P16 (22.5, -35.5)
  point P17 (22.5, -15.5)
  point P18 (22.5, -25.5)
  point P19 (20, -29)
  point P20 (22.5, -10.5)
  point P21 (22.5, -45.5)
  point P22 (25, -50)
  point P23 (20, -49)
  dimension "d90" = 2.5
  dimension "d91" = 2.5
  dimension "d92" = 2.5
  dimension "d93" = 2.5
  constraint coincident P10 L21.start
  constraint horizontal L13
  constraint coincident P9 L28
  constraint horizontal L18
  constraint coincident P1 L19
  constraint horizontal L37
  constraint coincident P4 L45
  constraint horizontal L17
  constraint coincident P3 L41
  constraint horizontal L39
  constraint coincident P6 L42
  constraint horizontal L12
  constraint coincident P2 L43
  constraint horizontal L44
  constraint coincident P5 L51
  constraint horizontal L15
  constraint coincident P8 L14
  constraint horizontal L26
  constraint coincident P0 L11
  constraint coincident P22 L68.start
  constraint horizontal L60
  constraint coincident P21 L75
  constraint horizontal L65
  constraint coincident P13 L66
  constraint horizontal L84
  constraint coincident P16 L92
  constraint horizontal L64
  constraint coincident P15 L88
  constraint horizontal L86
  constraint coincident P18 L89
  constraint horizontal L59
  constraint coincident P14 L90
  constraint horizontal L91
  constraint coincident P17 L98
  constraint horizontal L62
  constraint coincident P20 L61
  constraint horizontal L73
  constraint coincident P12 L58
  measures "d90" distance of P10 L21.end
  measures "d91" distance of L46.start L46.end
  measures "d92" distance of P22 L68.end
  measures "d93" distance of L93.start L93.end
extrude "Extrude14" cut sketch "Sketch12" sketch "Sketch13" against normal blind 105 contours L7 L37 L41 L50 | L8 L46 L51 L52 | L9 L18 L20 L33 | L10 L12 L27 L28 | L11 L15 L22 L25 | L14 L34 L35 L40 | L17 L29 L31 L32 | L19 L24 L38 L42 | L26 L36 L39 L49 of sketch 2 contours L7 L37 L41 L50 | L8 L46 L51 L52 | L9 L18 L20 L33 | L10 L12 L27 L28 | L11 L15 L22 L25 | L14 L34 L35 L40 | L17 L29 L31 L32 | L19 L24 L38 L42 | L26 L36 L39 L49 bodies 1
extrude "Extrude15" cut sketch "Sketch14" against normal blind 9 contours L5 L35 L39 L48 | L6 L44 L49 L50 | L7 L16 L18 L31 | L8 L10 L25 L26 | L9 L13 L20 L23 | L12 L32 L33 L38 | L15 L27 L29 L30 | L17 L22 L36 L40 | L24 L34 L37 L47 | L52 L82 L86 L95 | L53 L91 L96 L97 | L54 L63 L65 L78 | L55 L57 L72 L73 | L56 L60 L67 L70 | L59 L79 L80 L85 | L62 L74 L76 L77 | L64 L69 L83 L87 | L71 L81 L84 L94 bodies 1
sketch "Sketch15" plane through (20, 0, 0) normal (-1, 0, 0) x (0, -1, 0)
  line L0 (-100.5, -13.5) -> (-100.5, -17.5)
  line L1 (-100.5, -17.5) -> (-104.5, -17.5)
  line L2 (-104.5, -17.5) -> (-104.5, -13.5)
  line L3 (-104.5, -13.5) -> (-100.5, -13.5)
  line L4 (-100.5, -37.5) -> (-104.5, -37.5)
  line L5 (-104.5, -37.5) -> (-104.5, -33.5)
  line L6 (-104.5, -33.5) -> (-100.5, -33.5)
  line L7 (-100.5, -33.5) -> (-100.5, -37.5)
  line L8 (-100.5, -42.5) -> (-104.5, -42.5)
  line L9 (-104.5, -42.5) -> (-104.5, -38.5)
  line L10 (-104.5, -38.5) -> (-100.5, -38.5)
  line L11 (-100.5, -38.5) -> (-100.5, -42.5)
  line L12 (-104.5, -22.5) -> (-104.5, -18.5)
  line L13 (-104.5, -18.5) -> (-100.5, -18.5)
  line L14 (-100.5, -18.5) -> (-100.5, -22.5)
  line L15 (-100.5, -22.5) -> (-104.5, -22.5)
  line L16 (-100.5, -8.5) -> (-100.5, -12.5)
  line L17 (-100.5, -12.5) -> (-104.5, -12.5)
  line L18 (-104.5, -12.5) -> (-104.5, -8.5)
  line L19 (-104.5, -8.5) -> (-100.5, -8.5)
  line L20 (-100.5, -28.5) -> (-100.5, -32.5)
  line L21 (-100.5, -32.5) -> (-104.5, -32.5)
  line L22 (-104.5, -32.5) -> (-104.5, -28.5)
  line L23 (-104.5, -28.5) -> (-100.5, -28.5)
  line L24 (-100.5, -23.5) -> (-100.5, -27.5)
  line L25 (-100.5, -27.5) -> (-104.5, -27.5)
  line L26 (-104.5, -27.5) -> (-104.5, -23.5)
  line L27 (-104.5, -23.5) -> (-100.5, -23.5)
  line L28 (-104.5, -3.5) -> (-100.5, -3.5)
  line L29 (-100.5, -3.5) -> (-100.5, -7.5)
  line L30 (-100.5, -7.5) -> (-104.5, -7.5)
  line L31 (-104.5, -7.5) -> (-104.5, -3.5)
  line L32 (-100, -49) -> (-100, 0)
  line L33 (-100, 0) -> (-90, 0)
  line L34 (-90, 0) -> (-90, 3)
  line L35 (-90, 3) -> (-105, 3)
  line L36 (-105, 3) -> (-105, -50)
  line L37 (-105, -50) -> (-85, -50)
  line L38 (-85, -50) -> (-85, -49)
  line L39 (-85, -49) -> (-100, -49)
  line L40 (-104.5, -23.5) -> (-100.5, -23.5)
  line L41 (-104.5, -13.5) -> (-100.5, -13.5)
  line L42 (-100.5, -38.5) -> (-100.5, -42.5)
  line L43 (-100.5, -3.5) -> (-100.5, -7.5)
  line L44 (-100.5, -43.5) -> (-100.5, -47.5)
  line L45 (-104.5, -7.5) -> (-104.5, -3.5)
  line L46 (-100.5, -7.5) -> (-104.5, -3.5) construction
  line L47 (-100.5, -22.5) -> (-104.5, -22.5)
  line L48 (-100.5, -47.5) -> (-104.5, -47.5)
  line L49 (-100.5, -12.5) -> (-104.5, -8.5) construction
  line L50 (-100.5, -12.5) -> (-104.5, -12.5)
  line L51 (-104.5, -42.5) -> (-104.5, -38.5)
  line L52 (-100.5, -32.5) -> (-104.5, -32.5)
  line L53 (-100.5, -42.5) -> (-104.5, -42.5)
  line L54 (-100.5, -42.5) -> (-104.5, -38.5) construction
  line L55 (-104.5, -47.5) -> (-104.5, -43.5)
  line L56 (-100, -50) -> (-102.5, -50)
  line L57 (-100.5, -28.5) -> (-100.5, -32.5)
  line L58 (-104.5, -43.5) -> (-100.5, -43.5)
  line L59 (-104.5, -37.5) -> (-104.5, -33.5)
  line L60 (-104.5, -3.5) -> (-100.5, -3.5)
  line L61 (-100.5, -7.5) -> (-104.5, -7.5)
  line L62 (-104.5, -8.5) -> (-100.5, -8.5)
  line L63 (-100.5, -47.5) -> (-104.5, -43.5) construction
  line L64 (-100.5, -8.5) -> (-100.5, -12.5)
  line L65 (-104.5, -12.5) -> (-104.5, -8.5)
  line L66 (-104.5, -38.5) -> (-100.5, -38.5)
  line L67 (-104.5, -18.5) -> (-100.5, -18.5)
  line L68 (-104.5, -22.5) -> (-104.5, -18.5)
  line L69 (-100.5, -33.5) -> (-100.5, -37.5)
  line L70 (-100.5, -23.5) -> (-100.5, -27.5)
  line L71 (-104.5, -28.5) -> (-100.5, -28.5)
  line L72 (-100.5, -37.5) -> (-104.5, -37.5)
  line L73 (-100.5, -18.5) -> (-100.5, -22.5)
  line L74 (-100.5, -27.5) -> (-104.5, -27.5)
  line L75 (-104.5, -32.5) -> (-104.5, -28.5)
  line L76 (-100.5, -32.5) -> (-104.5, -28.5) construction
  line L77 (-100.5, -27.5) -> (-104.5, -23.5) construction
  line L78 (-100.5, -22.5) -> (-104.5, -18.5) construction
  line L79 (-100.5, -17.5) -> (-104.5, -17.5)
  line L80 (-100.5, -37.5) -> (-104.5, -33.5) construction
  line L81 (-100, -30) -> (-102.5, -30)
  line L82 (-104.5, -33.5) -> (-100.5, -33.5)
  line L83 (-104.5, -27.5) -> (-104.5, -23.5)
  line L84 (-100.5, -13.5) -> (-100.5, -17.5)
  line L85 (-104.5, -17.5) -> (-104.5, -13.5)
  line L86 (-100.5, -17.5) -> (-104.5, -13.5) construction
  point P0 (-102.5, -5.5)
  point P1 (-102.5, -40.5)
  point P2 (-102.5, -20.5)
  point P3 (-102.5, -30.5)
  point P4 (-102.5, -35.5)
  point P5 (-102.5, -15.5)
  point P6 (-102.5, -25.5)
  point P7 (-105, -29)
  point P8 (-102.5, -10.5)
  point P9 (-102.5, -45.5)
  point P10 (-100, -50)
  point P11 (-105, -49)
  dimension "d98" = 2.5
  dimension "d99" = 2.5
  constraint coincident P10 L56.start
  constraint horizontal L48
  constraint coincident P9 L63
  constraint horizontal L53
  constraint coincident P1 L54
  constraint horizontal L72
  constraint coincident P4 L80
  constraint horizontal L52
  constraint coincident P3 L76
  constraint horizontal L74
  constraint coincident P6 L77
  constraint horizontal L47
  constraint coincident P2 L78
  constraint horizontal L79
  constraint coincident P5 L86
  constraint horizontal L50
  constraint coincident P8 L49
  constraint horizontal L61
  constraint coincident P0 L46
  measures "d98" distance of P10 L56.end
  measures "d99" distance of L81.start L81.end
extrude "Extrude16" cut sketch "Sketch15" against normal blind 10 contours L44 L48 L55 L58 bodies 1
sketch "Sketch16" plane through (80, 0, 0) normal (1, 0, 0) x (0, 1, 0)
  line L0 (100.5, -17.5) -> (100.5, -13.5)
  line L1 (100.5, -13.5) -> (104.5, -13.5)
  line L2 (104.5, -13.5) -> (104.5, -17.5)
  line L3 (104.5, -17.5) -> (100.5, -17.5)
  line L4 (104.5, -37.5) -> (100.5, -37.5)
  line L5 (100.5, -37.5) -> (100.5, -33.5)
  line L6 (100.5, -33.5) -> (104.5, -33.5)
  line L7 (104.5, -33.5) -> (104.5, -37.5)
  line L8 (104.5, -42.5) -> (100.5, -42.5)
  line L9 (100.5, -42.5) -> (100.5, -38.5)
  line L10 (100.5, -38.5) -> (104.5, -38.5)
  line L11 (104.5, -38.5) -> (104.5, -42.5)
  line L12 (104.5, -18.5) -> (104.5, -22.5)
  line L13 (104.5, -22.5) -> (100.5, -22.5)
  line L14 (100.5, -22.5) -> (100.5, -18.5)
  line L15 (100.5, -18.5) -> (104.5, -18.5)
  line L16 (100.5, -12.5) -> (100.5, -8.5)
  line L17 (100.5, -8.5) -> (104.5, -8.5)
  line L18 (104.5, -8.5) -> (104.5, -12.5)
  line L19 (104.5, -12.5) -> (100.5, -12.5)
  line L20 (100.5, -32.5) -> (100.5, -28.5)
  line L21 (100.5, -28.5) -> (104.5, -28.5)
  line L22 (104.5, -28.5) -> (104.5, -32.5)
  line L23 (104.5, -32.5) -> (100.5, -32.5)
  line L24 (100.5, -27.5) -> (100.5, -23.5)
  line L25 (100.5, -23.5) -> (104.5, -23.5)
  line L26 (104.5, -23.5) -> (104.5, -27.5)
  line L27 (104.5, -27.5) -> (100.5, -27.5)
  line L28 (100.5, -3.5) -> (104.5, -3.5)
  line L29 (104.5, -3.5) -> (104.5, -7.5)
  line L30 (104.5, -7.5) -> (100.5, -7.5)
  line L31 (100.5, -7.5) -> (100.5, -3.5)
  line L32 (105, -50) -> (105, 3)
  line L33 (105, 3) -> (90, 3)
  line L34 (90, 3) -> (90, 0)
  line L35 (90, 0) -> (100, 0)
  line L36 (100, 0) -> (100, -49)
  line L37 (100, -49) -> (85, -49)
  line L38 (85, -49) -> (85, -50)
  line L39 (85, -50) -> (105, -50)
  line L40 (100.5, -38.5) -> (104.5, -38.5)
  line L41 (104.5, -38.5) -> (104.5, -42.5)
  line L42 (104.5, -42.5) -> (100.5, -42.5)
  line L43 (100.5, -42.5) -> (100.5, -38.5)
  line L44 (100.5, -43.5) -> (104.5, -43.5)
  line L45 (104.5, -43.5) -> (104.5, -47.5)
  line L46 (104.5, -47.5) -> (100.5, -47.5)
  line L47 (100.5, -47.5) -> (100.5, -43.5)
extrude "Extrude17" cut sketch "Sketch16" against normal blind 7 contours L44 L45 L46 L47 bodies 1
sketch "Sketch17" plane through (0, 0, -49) normal (0, 0, 1) x (-1, 0, 0)
  line L0 (-35, -75) -> (-35, -105)
  line L1 (-35, -105) -> (-25, -105)
  line L2 (-25, -105) -> (-25, -100)
  line L3 (-25, -100) -> (-20, -100)
  line L4 (-20, -100) -> (-20, -85)
  line L5 (-20, -85) -> (5, -60)
  line L6 (5, -60) -> (5, 0)
  line L7 (5, 0) -> (0, 0)
  line L8 (0, 0) -> (0, 5)
  line L9 (0, 5) -> (-100, 5)
  line L10 (-100, 5) -> (-100, 0)
  line L11 (-100, 0) -> (-105, 0)
  line L12 (-105, 0) -> (-105, -60)
  line L13 (-105, -60) -> (-80, -85)
  line L14 (-80, -85) -> (-80, -100)
  line L15 (-80, -100) -> (-75, -100)
  line L16 (-75, -100) -> (-75, -105)
  line L17 (-75, -105) -> (-65, -105)
  line L18 (-65, -105) -> (-65, -75)
  line L19 (-65, -75) -> (-35, -75)
  line L20 (5, 5) -> (5, -60)
  line L21 (5, -60) -> (-20, -85)
  line L22 (-20, -85) -> (-20, -105)
  line L23 (-20, -105) -> (-80, -105)
  line L24 (-80, -105) -> (-80, -85)
  line L25 (-80, -85) -> (-105, -60)
  line L26 (-105, -60) -> (-105, 5)
  line L27 (-105, 5) -> (5, 5)
  line L28 (5, 5) -> (4, 5)
  line L29 (-20, -105) -> (-21, -105)
  line L30 (-80, -105) -> (-80, -104)
  line L31 (-80, -104) -> (-21, -104)
  line L32 (-80, -104) -> (-79, -104)
  line L33 (-79, -104) -> (-79, -85)
  line L34 (-79, -85) -> (-104, -60)
  line L35 (-104, -60) -> (-104, 4)
  line L36 (-104, 4) -> (4, 4)
  line L37 (4, 4) -> (4, -60)
  line L38 (4, -60) -> (-21, -85)
  line L39 (-21, -85) -> (-21, -104)
  line L40 (-35, -104) -> (-65, -104)
  line L41 (-65, -104) -> (-65, -105)
  line L42 (-65, -105) -> (-35, -105)
  line L43 (-35, -105) -> (-35, -104)
  dimension "d104" = 1
  dimension "d106" = 1
  dimension "d107" = 1
  dimension "d108" = 19
  dimension "d109" = 64
  constraint coincident L5.end L6.start
  constraint coincident L4.end L5.start
  constraint coincident L13.end L14.start
  constraint perpendicular L23 L24
  constraint coincident L12.end L13.start
  constraint perpendicular L20 L28
  constraint coincident L23 L29.end
  constraint perpendicular L22 L29
  constraint perpendicular L23 L30
  constraint coincident L31 L32.end
  constraint perpendicular L24 L32
  constraint perpendicular L32 L33
  constraint perpendicular L11 L35
  constraint perpendicular L36 L37
  constraint coincident L31 L40.start
  constraint coincident L0 L40.start
  constraint coincident L31 L40.end
  constraint coincident L18 L40.end
  constraint coincident L17.end L18.start
  constraint coincident L0.end L1.start
  measures "d104" distance of L20.start L28.end
  measures "d106" distance of L22.end L29.end
  measures "d107" distance of L23.end L30.end
  measures "d108" distance of L32.end L33.end
  measures "d109" distance of L34.end L35.end
extrude "Extrude18" add sketch "Sketch17" along normal blind 2.5 contours L0 L1 L2 L23 L31 L43 | L16 L17 L18 L23 L31 L41 | L3 L4 L5 L6 L7 L20 L21 L22 L37 L38 L39 | L11 L12 L13 L14 L15 L24 L25 L26 L33 L34 L35 | L8 L9 L10 L27 L36 bodies 1
move_body "Move1" bodies 1 to x (1, 0, 0) y (0, 1, 0) z (0, 0, 1) at (0, 0, 50)
ref_plane "WorkPlane2" through (96.5, 3.5, 50) normal (-0.707107, -0.707107, 0) x (0.707107, -0.707107, 0)
ref_plane "WorkPlane3" through (71.5, 96.5, 50) normal (0.707107, -0.707107, 0) x (0.707107, 0.707107, 0)
ref_plane "WorkPlane4" through (25, 100, 50) normal (0.707107, 0.707107, 0) x (-0.707107, 0.707107, 0)
ref_plane "WorkPlane5" through (3.5, 3.5, 50) normal (-0.707107, 0.707107, 0) x (-0.707107, -0.707107, 0)
sketch "Sketch18" plane through (50, 50, 0) normal (-0.707107, -0.707107, 0) x (0.707107, -0.707107, 0)
sketch "Sketch19" plane through (-12.5, 12.5, 0) normal (0.707107, -0.707107, 0) x (0.707107, 0.707107, 0)
